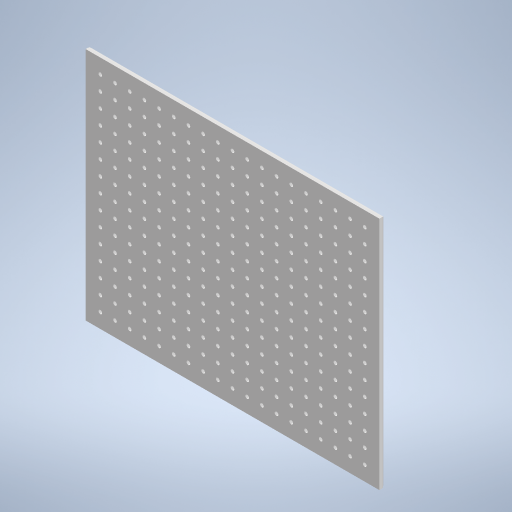
# Autodesk Inventor part: attachments_hub
Saved by Autodesk Inventor 2024.3 (Build 283343000, 343)
## iProperties
Created: 2026-05-03
Part Number: attachments_hub
Material: Generic
Document SubType Name: Modeling
Designer: owozn
Density: 1 g/cm^3
Appearance: Default
Author: owozn
Autodesk Inventor part; units mm, degrees
ref_plane "YZ Plane" through (0, 0, 0) normal (1, 0, 0) x (0, 1, 0)
ref_plane "XZ Plane" through (0, 0, 0) normal (0, 1, 0) x (-1, 0, 0)
ref_plane "XY Plane" through (0, 0, 0) normal (0, 0, 1) x (1, 0, 0)
ref_plane "Work Plane1" through (-31.4326, 14.9861, 0) normal (0, 0, 1) x (1, 0, 0)
sketch "Sketch1" plane through (-31.4326, 14.9861, 0) normal (0, 0, 1) x (1, 0, 0)
  line L0 (31.4326, -44.9861) -> (31.4326, 25.0139) projected
  line L1 (-16.1674, -14.9861) -> (79.0326, -14.9861) projected
  line L2 (-2.5674, 15.0139) -> (7.4326, 15.0139)
  line L3 (7.4326, 15.0139) -> (7.4326, -34.9861)
  line L4 (7.4326, -34.9861) -> (-2.5674, -34.9861)
  line L5 (-2.5674, -34.9861) -> (-2.5674, 15.0139)
  line L6 (-2.5674, 15.0139) -> (7.4326, -34.9861) construction
  line L7 (7.4326, 15.0139) -> (-2.5674, -34.9861) construction
  line L8 (65.4326, 15.0139) -> (55.4326, 15.0139)
  line L9 (55.4326, 15.0139) -> (55.4326, -34.9861)
  line L10 (55.4326, -34.9861) -> (65.4326, -34.9861)
  line L11 (65.4326, -34.9861) -> (65.4326, 15.0139)
  line L12 (65.4326, 15.0139) -> (55.4326, -34.9861) construction
  line L13 (55.4326, 15.0139) -> (65.4326, -34.9861) construction
  point P0 (31.4326, -14.9861)
  point P1 (2.4326, -9.9861)
  point P2 (60.4326, -9.9861)
  dimension "d0" = 10
  dimension "d1" = 50
  dimension "d2" = 29
  dimension "d3" = 5
  constraints: 24 end point, 5 symmetric about line, 2 midpoint, 2 parallel, 1 horizontal, 1 perpendicular
  measures "d0" distance of L3.end L4.end
  measures "d1" distance of L2.end L3.end
  measures "d2" distance from line of L0 point (2.433, -9.986)
  measures "d3" distance from line of L1 point (2.433, -9.986)
extrude "Extrusion1" add sketch "Sketch1" along normal blind 35
sketch "Sketch2" plane through (24, -20, 0) normal (-1, 0, 0) x (0, 0, 1)
  line L0 (0, -10) -> (0, 60) projected
  line L1 (-7, 20) -> (42, 20) projected
  circle A0 centre (7, 25) radius 1.6
  circle A1 centre (7, 41) radius 1.6
  line L2 (8.6, 25) -> (8.6, 41)
  line L3 (5.4, 25) -> (5.4, 41)
  point P0 (0, 20)
  dimension "d6" = 3.2
  dimension "d7" = 3.2
  dimension "d8" = 7
  dimension "d9" = 7
  dimension "d10" = 21
  dimension "d11" = 5
  constraints: 4 end point, 4 point on circle, 4 tangent, 2 centre point
  measures "d6" diameter of A0
  measures "d7" diameter of A1
  measures "d8" distance from line of L0 A0.centre
  measures "d9" distance from line of L0 A1.centre
  measures "d10" distance from line of L1 A1.centre
  measures "d11" distance from line of L1 A0.centre
extrude "Extrusion2" cut sketch "Sketch2" along normal through all both and the other way through all
sketch "Sketch3" plane through (-31.4326, 14.9861, 35) normal (0, 0, 1) x (1, 0, 0)
  line L0 (31.4326, -154.9861) -> (31.4326, 125.0139) projected
  line L1 (-152.3174, -14.9861) -> (215.1826, -14.9861) projected
  line L2 (156.4326, -114.9861) -> (-93.5674, -114.9861)
  line L3 (-93.5674, -114.9861) -> (-93.5674, 85.0139)
  line L4 (-93.5674, 85.0139) -> (156.4326, 85.0139)
  line L5 (156.4326, 85.0139) -> (156.4326, -114.9861)
  line L6 (156.4326, -114.9861) -> (-93.5674, 85.0139) construction
  line L7 (-93.5674, -114.9861) -> (156.4326, 85.0139) construction
  circle A0 centre (-81.0674, 72.5139) radius 1.6
  circle A1 centre (-68.5674, 72.5139) radius 1.6
  circle A2 centre (-56.0674, 72.5139) radius 1.6
  circle A3 centre (-43.5674, 72.5139) radius 1.6
  circle A4 centre (-31.0674, 72.5139) radius 1.6
  circle A5 centre (-18.5674, 72.5139) radius 1.6
  circle A6 centre (-6.0674, 72.5139) radius 1.6
  circle A7 centre (6.4326, 72.5139) radius 1.6
  circle A8 centre (18.9326, 72.5139) radius 1.6
  circle A9 centre (31.4326, 72.5139) radius 1.6
  circle A10 centre (43.9326, 72.5139) radius 1.6
  circle A11 centre (56.4326, 72.5139) radius 1.6
  circle A12 centre (68.9326, 72.5139) radius 1.6
  circle A13 centre (81.4326, 72.5139) radius 1.6
  circle A14 centre (93.9326, 72.5139) radius 1.6
  circle A15 centre (106.4326, 72.5139) radius 1.6
  circle A16 centre (118.9326, 72.5139) radius 1.6
  circle A17 centre (131.4326, 72.5139) radius 1.6
  circle A18 centre (143.9326, 72.5139) radius 1.6
  circle A19 centre (-81.0674, 60.0139) radius 1.6
  circle A20 centre (-68.5674, 60.0139) radius 1.6
  circle A21 centre (-56.0674, 60.0139) radius 1.6
  circle A22 centre (-43.5674, 60.0139) radius 1.6
  circle A23 centre (-31.0674, 60.0139) radius 1.6
  circle A24 centre (-18.5674, 60.0139) radius 1.6
  circle A25 centre (-6.0674, 60.0139) radius 1.6
  circle A26 centre (6.4326, 60.0139) radius 1.6
  circle A27 centre (18.9326, 60.0139) radius 1.6
  circle A28 centre (31.4326, 60.0139) radius 1.6
  circle A29 centre (43.9326, 60.0139) radius 1.6
  circle A30 centre (56.4326, 60.0139) radius 1.6
  circle A31 centre (68.9326, 60.0139) radius 1.6
  circle A32 centre (81.4326, 60.0139) radius 1.6
  circle A33 centre (93.9326, 60.0139) radius 1.6
  circle A34 centre (106.4326, 60.0139) radius 1.6
  circle A35 centre (118.9326, 60.0139) radius 1.6
  circle A36 centre (131.4326, 60.0139) radius 1.6
  circle A37 centre (143.9326, 60.0139) radius 1.6
  circle A38 centre (-81.0674, 47.5139) radius 1.6
  circle A39 centre (-68.5674, 47.5139) radius 1.6
  circle A40 centre (-56.0674, 47.5139) radius 1.6
  circle A41 centre (-43.5674, 47.5139) radius 1.6
  circle A42 centre (-31.0674, 47.5139) radius 1.6
  circle A43 centre (-18.5674, 47.5139) radius 1.6
  circle A44 centre (-6.0674, 47.5139) radius 1.6
  circle A45 centre (6.4326, 47.5139) radius 1.6
  circle A46 centre (18.9326, 47.5139) radius 1.6
  circle A47 centre (31.4326, 47.5139) radius 1.6
  circle A48 centre (43.9326, 47.5139) radius 1.6
  circle A49 centre (56.4326, 47.5139) radius 1.6
  circle A50 centre (68.9326, 47.5139) radius 1.6
  circle A51 centre (81.4326, 47.5139) radius 1.6
  circle A52 centre (93.9326, 47.5139) radius 1.6
  circle A53 centre (106.4326, 47.5139) radius 1.6
  circle A54 centre (118.9326, 47.5139) radius 1.6
  circle A55 centre (131.4326, 47.5139) radius 1.6
  circle A56 centre (143.9326, 47.5139) radius 1.6
  circle A57 centre (-81.0674, 35.0139) radius 1.6
  circle A58 centre (-68.5674, 35.0139) radius 1.6
  circle A59 centre (-56.0674, 35.0139) radius 1.6
  circle A60 centre (-43.5674, 35.0139) radius 1.6
  circle A61 centre (-31.0674, 35.0139) radius 1.6
  circle A62 centre (-18.5674, 35.0139) radius 1.6
  circle A63 centre (-6.0674, 35.0139) radius 1.6
  circle A64 centre (6.4326, 35.0139) radius 1.6
  circle A65 centre (18.9326, 35.0139) radius 1.6
  circle A66 centre (31.4326, 35.0139) radius 1.6
  circle A67 centre (43.9326, 35.0139) radius 1.6
  circle A68 centre (56.4326, 35.0139) radius 1.6
  circle A69 centre (68.9326, 35.0139) radius 1.6
  circle A70 centre (81.4326, 35.0139) radius 1.6
  circle A71 centre (93.9326, 35.0139) radius 1.6
  circle A72 centre (106.4326, 35.0139) radius 1.6
  circle A73 centre (118.9326, 35.0139) radius 1.6
  circle A74 centre (131.4326, 35.0139) radius 1.6
  circle A75 centre (143.9326, 35.0139) radius 1.6
  circle A76 centre (-81.0674, 22.5139) radius 1.6
  circle A77 centre (-68.5674, 22.5139) radius 1.6
  circle A78 centre (-56.0674, 22.5139) radius 1.6
  circle A79 centre (-43.5674, 22.5139) radius 1.6
  circle A80 centre (-31.0674, 22.5139) radius 1.6
  circle A81 centre (-18.5674, 22.5139) radius 1.6
  circle A82 centre (-6.0674, 22.5139) radius 1.6
  circle A83 centre (6.4326, 22.5139) radius 1.6
  circle A84 centre (18.9326, 22.5139) radius 1.6
  circle A85 centre (31.4326, 22.5139) radius 1.6
  circle A86 centre (43.9326, 22.5139) radius 1.6
  circle A87 centre (56.4326, 22.5139) radius 1.6
  circle A88 centre (68.9326, 22.5139) radius 1.6
  circle A89 centre (81.4326, 22.5139) radius 1.6
  circle A90 centre (93.9326, 22.5139) radius 1.6
  circle A91 centre (106.4326, 22.5139) radius 1.6
  circle A92 centre (118.9326, 22.5139) radius 1.6
  circle A93 centre (131.4326, 22.5139) radius 1.6
  circle A94 centre (143.9326, 22.5139) radius 1.6
  circle A95 centre (-81.0674, 10.0139) radius 1.6
  circle A96 centre (-68.5674, 10.0139) radius 1.6
  circle A97 centre (-56.0674, 10.0139) radius 1.6
  circle A98 centre (-43.5674, 10.0139) radius 1.6
  circle A99 centre (-31.0674, 10.0139) radius 1.6
  circle A100 centre (-18.5674, 10.0139) radius 1.6
  circle A101 centre (-6.0674, 10.0139) radius 1.6
  circle A102 centre (6.4326, 10.0139) radius 1.6
  circle A103 centre (18.9326, 10.0139) radius 1.6
  circle A104 centre (31.4326, 10.0139) radius 1.6
  circle A105 centre (43.9326, 10.0139) radius 1.6
  circle A106 centre (56.4326, 10.0139) radius 1.6
  circle A107 centre (68.9326, 10.0139) radius 1.6
  circle A108 centre (81.4326, 10.0139) radius 1.6
  circle A109 centre (93.9326, 10.0139) radius 1.6
  circle A110 centre (106.4326, 10.0139) radius 1.6
  circle A111 centre (118.9326, 10.0139) radius 1.6
  circle A112 centre (131.4326, 10.0139) radius 1.6
  circle A113 centre (143.9326, 10.0139) radius 1.6
  circle A114 centre (-81.0674, -2.4861) radius 1.6
  circle A115 centre (-68.5674, -2.4861) radius 1.6
  circle A116 centre (-56.0674, -2.4861) radius 1.6
  circle A117 centre (-43.5674, -2.4861) radius 1.6
  circle A118 centre (-31.0674, -2.4861) radius 1.6
  circle A119 centre (-18.5674, -2.4861) radius 1.6
  circle A120 centre (-6.0674, -2.4861) radius 1.6
  circle A121 centre (6.4326, -2.4861) radius 1.6
  circle A122 centre (18.9326, -2.4861) radius 1.6
  circle A123 centre (31.4326, -2.4861) radius 1.6
  circle A124 centre (43.9326, -2.4861) radius 1.6
  circle A125 centre (56.4326, -2.4861) radius 1.6
  circle A126 centre (68.9326, -2.4861) radius 1.6
  circle A127 centre (81.4326, -2.4861) radius 1.6
  circle A128 centre (93.9326, -2.4861) radius 1.6
  circle A129 centre (106.4326, -2.4861) radius 1.6
  circle A130 centre (118.9326, -2.4861) radius 1.6
  circle A131 centre (131.4326, -2.4861) radius 1.6
  circle A132 centre (143.9326, -2.4861) radius 1.6
  circle A133 centre (-81.0674, -14.9861) radius 1.6
  circle A134 centre (-68.5674, -14.9861) radius 1.6
  circle A135 centre (-56.0674, -14.9861) radius 1.6
  circle A136 centre (-43.5674, -14.9861) radius 1.6
  circle A137 centre (-31.0674, -14.9861) radius 1.6
  circle A138 centre (-18.5674, -14.9861) radius 1.6
  circle A139 centre (-6.0674, -14.9861) radius 1.6
  circle A140 centre (6.4326, -14.9861) radius 1.6
  circle A141 centre (18.9326, -14.9861) radius 1.6
  circle A142 centre (31.4326, -14.9861) radius 1.6
  circle A143 centre (43.9326, -14.9861) radius 1.6
  circle A144 centre (56.4326, -14.9861) radius 1.6
  circle A145 centre (68.9326, -14.9861) radius 1.6
  circle A146 centre (81.4326, -14.9861) radius 1.6
  circle A147 centre (93.9326, -14.9861) radius 1.6
  circle A148 centre (106.4326, -14.9861) radius 1.6
  circle A149 centre (118.9326, -14.9861) radius 1.6
  circle A150 centre (131.4326, -14.9861) radius 1.6
  circle A151 centre (143.9326, -14.9861) radius 1.6
  circle A152 centre (-81.0674, -27.4861) radius 1.6
  circle A153 centre (-68.5674, -27.4861) radius 1.6
  circle A154 centre (-56.0674, -27.4861) radius 1.6
  circle A155 centre (-43.5674, -27.4861) radius 1.6
  circle A156 centre (-31.0674, -27.4861) radius 1.6
  circle A157 centre (-18.5674, -27.4861) radius 1.6
  circle A158 centre (-6.0674, -27.4861) radius 1.6
  circle A159 centre (6.4326, -27.4861) radius 1.6
  circle A160 centre (18.9326, -27.4861) radius 1.6
  circle A161 centre (31.4326, -27.4861) radius 1.6
  circle A162 centre (43.9326, -27.4861) radius 1.6
  circle A163 centre (56.4326, -27.4861) radius 1.6
  circle A164 centre (68.9326, -27.4861) radius 1.6
  circle A165 centre (81.4326, -27.4861) radius 1.6
  circle A166 centre (93.9326, -27.4861) radius 1.6
  circle A167 centre (106.4326, -27.4861) radius 1.6
  circle A168 centre (118.9326, -27.4861) radius 1.6
  circle A169 centre (131.4326, -27.4861) radius 1.6
  circle A170 centre (143.9326, -27.4861) radius 1.6
  circle A171 centre (-81.0674, -39.9861) radius 1.6
  circle A172 centre (-68.5674, -39.9861) radius 1.6
  circle A173 centre (-56.0674, -39.9861) radius 1.6
  circle A174 centre (-43.5674, -39.9861) radius 1.6
  circle A175 centre (-31.0674, -39.9861) radius 1.6
  circle A176 centre (-18.5674, -39.9861) radius 1.6
  circle A177 centre (-6.0674, -39.9861) radius 1.6
  circle A178 centre (6.4326, -39.9861) radius 1.6
  circle A179 centre (18.9326, -39.9861) radius 1.6
  circle A180 centre (31.4326, -39.9861) radius 1.6
  circle A181 centre (43.9326, -39.9861) radius 1.6
  circle A182 centre (56.4326, -39.9861) radius 1.6
  circle A183 centre (68.9326, -39.9861) radius 1.6
  circle A184 centre (81.4326, -39.9861) radius 1.6
  circle A185 centre (93.9326, -39.9861) radius 1.6
  circle A186 centre (106.4326, -39.9861) radius 1.6
  circle A187 centre (118.9326, -39.9861) radius 1.6
  circle A188 centre (131.4326, -39.9861) radius 1.6
  circle A189 centre (143.9326, -39.9861) radius 1.6
  circle A190 centre (-81.0674, -52.4861) radius 1.6
  circle A191 centre (-68.5674, -52.4861) radius 1.6
  circle A192 centre (-56.0674, -52.4861) radius 1.6
  circle A193 centre (-43.5674, -52.4861) radius 1.6
  circle A194 centre (-31.0674, -52.4861) radius 1.6
  circle A195 centre (-18.5674, -52.4861) radius 1.6
  circle A196 centre (-6.0674, -52.4861) radius 1.6
  circle A197 centre (6.4326, -52.4861) radius 1.6
  circle A198 centre (18.9326, -52.4861) radius 1.6
  circle A199 centre (31.4326, -52.4861) radius 1.6
  circle A200 centre (43.9326, -52.4861) radius 1.6
  circle A201 centre (56.4326, -52.4861) radius 1.6
  circle A202 centre (68.9326, -52.4861) radius 1.6
  circle A203 centre (81.4326, -52.4861) radius 1.6
  circle A204 centre (93.9326, -52.4861) radius 1.6
  circle A205 centre (106.4326, -52.4861) radius 1.6
  circle A206 centre (118.9326, -52.4861) radius 1.6
  circle A207 centre (131.4326, -52.4861) radius 1.6
  circle A208 centre (143.9326, -52.4861) radius 1.6
  circle A209 centre (-81.0674, -64.9861) radius 1.6
  circle A210 centre (-68.5674, -64.9861) radius 1.6
  circle A211 centre (-56.0674, -64.9861) radius 1.6
  circle A212 centre (-43.5674, -64.9861) radius 1.6
  circle A213 centre (-31.0674, -64.9861) radius 1.6
  circle A214 centre (-18.5674, -64.9861) radius 1.6
  circle A215 centre (-6.0674, -64.9861) radius 1.6
  circle A216 centre (6.4326, -64.9861) radius 1.6
  circle A217 centre (18.9326, -64.9861) radius 1.6
  circle A218 centre (31.4326, -64.9861) radius 1.6
  circle A219 centre (43.9326, -64.9861) radius 1.6
  circle A220 centre (56.4326, -64.9861) radius 1.6
  circle A221 centre (68.9326, -64.9861) radius 1.6
  circle A222 centre (81.4326, -64.9861) radius 1.6
  circle A223 centre (93.9326, -64.9861) radius 1.6
  circle A224 centre (106.4326, -64.9861) radius 1.6
  circle A225 centre (118.9326, -64.9861) radius 1.6
  circle A226 centre (131.4326, -64.9861) radius 1.6
  circle A227 centre (143.9326, -64.9861) radius 1.6
  circle A228 centre (-81.0674, -77.4861) radius 1.6
  circle A229 centre (-68.5674, -77.4861) radius 1.6
  circle A230 centre (-56.0674, -77.4861) radius 1.6
  circle A231 centre (-43.5674, -77.4861) radius 1.6
  circle A232 centre (-31.0674, -77.4861) radius 1.6
  circle A233 centre (-18.5674, -77.4861) radius 1.6
  circle A234 centre (-6.0674, -77.4861) radius 1.6
  circle A235 centre (6.4326, -77.4861) radius 1.6
  circle A236 centre (18.9326, -77.4861) radius 1.6
  circle A237 centre (31.4326, -77.4861) radius 1.6
  circle A238 centre (43.9326, -77.4861) radius 1.6
  circle A239 centre (56.4326, -77.4861) radius 1.6
  circle A240 centre (68.9326, -77.4861) radius 1.6
  circle A241 centre (81.4326, -77.4861) radius 1.6
  circle A242 centre (93.9326, -77.4861) radius 1.6
  circle A243 centre (106.4326, -77.4861) radius 1.6
  circle A244 centre (118.9326, -77.4861) radius 1.6
  circle A245 centre (131.4326, -77.4861) radius 1.6
  circle A246 centre (143.9326, -77.4861) radius 1.6
  circle A247 centre (-81.0674, -89.9861) radius 1.6
  circle A248 centre (-68.5674, -89.9861) radius 1.6
  circle A249 centre (-56.0674, -89.9861) radius 1.6
  circle A250 centre (-43.5674, -89.9861) radius 1.6
  circle A251 centre (-31.0674, -89.9861) radius 1.6
  circle A252 centre (-18.5674, -89.9861) radius 1.6
  circle A253 centre (-6.0674, -89.9861) radius 1.6
  circle A254 centre (6.4326, -89.9861) radius 1.6
  circle A255 centre (18.9326, -89.9861) radius 1.6
  circle A256 centre (31.4326, -89.9861) radius 1.6
  circle A257 centre (43.9326, -89.9861) radius 1.6
  circle A258 centre (56.4326, -89.9861) radius 1.6
  circle A259 centre (68.9326, -89.9861) radius 1.6
  circle A260 centre (81.4326, -89.9861) radius 1.6
  circle A261 centre (93.9326, -89.9861) radius 1.6
  circle A262 centre (106.4326, -89.9861) radius 1.6
  circle A263 centre (118.9326, -89.9861) radius 1.6
  circle A264 centre (131.4326, -89.9861) radius 1.6
  circle A265 centre (143.9326, -89.9861) radius 1.6
  circle A266 centre (-81.0674, -102.4861) radius 1.6
  circle A267 centre (-68.5674, -102.4861) radius 1.6
  circle A268 centre (-56.0674, -102.4861) radius 1.6
  circle A269 centre (-43.5674, -102.4861) radius 1.6
  circle A270 centre (-31.0674, -102.4861) radius 1.6
  circle A271 centre (-18.5674, -102.4861) radius 1.6
  circle A272 centre (-6.0674, -102.4861) radius 1.6
  circle A273 centre (6.4326, -102.4861) radius 1.6
  circle A274 centre (18.9326, -102.4861) radius 1.6
  circle A275 centre (31.4326, -102.4861) radius 1.6
  circle A276 centre (43.9326, -102.4861) radius 1.6
  circle A277 centre (56.4326, -102.4861) radius 1.6
  circle A278 centre (68.9326, -102.4861) radius 1.6
  circle A279 centre (81.4326, -102.4861) radius 1.6
  circle A280 centre (93.9326, -102.4861) radius 1.6
  circle A281 centre (106.4326, -102.4861) radius 1.6
  circle A282 centre (118.9326, -102.4861) radius 1.6
  circle A283 centre (131.4326, -102.4861) radius 1.6
  circle A284 centre (143.9326, -102.4861) radius 1.6
  point P0 (31.4326, -14.9861)
  dimension "d14" = 250
  dimension "d15" = 200
  dimension "d19" = 3.2
  dimension "d20" = 12.5
  dimension "d21" = 12.5
  dimension "d24" = 12.5
  dimension "d27" = 12.5
  constraints: 285 centre point, 12 end point, 2 horizontal, 2 midpoint, 2 parallel, 1 perpendicular, 1 vertical, 568 other
  measures "d14" distance of L3.end L4.end
  measures "d15" distance of L2.end L3.end
  measures "d19" diameter of A0
  measures "d20" distance from line of L4 A0.centre
  measures "d21" distance from line of L3 A0.centre
  measures "d24" distance of A0.centre A1.centre
  measures "d27" distance of A0.centre A19.centre
extrude "Extrusion3" add sketch "Sketch3" along normal blind 5 contours L2 L3 L1 A133 A134 A135 A136 A137 A138 A139 A140 A141 A142 L0 A161 A180 A199 A218 A237 A256 A275 | L0 A275 A256 A237 A218 A199 A180 A161 A142 L1 A143 A144 A145 A146 A147 A148 A149 A150 A151 L5 L2 | L1 A151 A150 A149 A148 A147 A146 A145 A144 A143 A142 L0 A123 A104 A85 A66 A47 A28 A9 L4 L5 | L3 L4 L0 A9 A28 A47 A66 A85 A104 A123 A142 L1 A141 A140 A139 A138 A137 A136 A135 A134 A133
fillet "Fillet2" radius 3 12 edges at (-24, -20, 17.5) (-34, -20, 17.5) (-34, 30, 17.5) (-24, 30, 17.5) (24, -20, 17.5) (24, 30, 17.5) (34, 30, 17.5) (34, -20, 17.5) (0, -100, 35) (125, 0, 35) (0, 100, 35) (-125, 0, 35)
body "Solid1"
